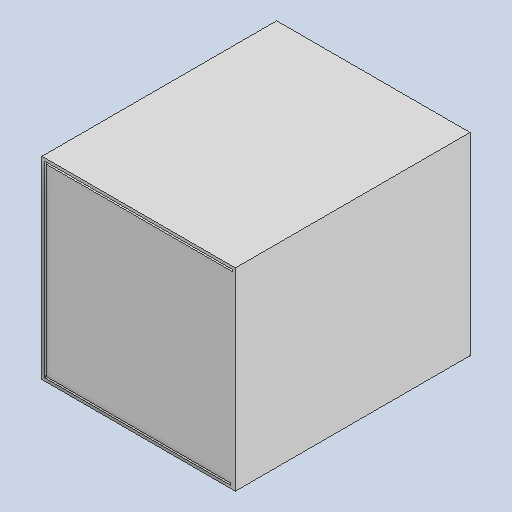
# Autodesk Inventor part: Envolvente
Saved by Autodesk Inventor 2024 (Build 280153000, 153)
## iProperties
Created: 2024-07-16
Part Number: Envolvente
Material: Genérico
Document SubType Name: Modeling
Designer: sergi
Density: 1 g/cm^3
Appearance: Valor por defecto
Author: sergi
Autodesk Inventor part; units mm, degrees
ref_plane "YZ Plane" through (0, 0, 0) normal (1, 0, 0) x (0, 1, 0)
ref_plane "XZ Plane" through (0, 0, 0) normal (0, 1, 0) x (-1, 0, 0)
ref_plane "XY Plane" through (0, 0, 0) normal (0, 0, 1) x (1, 0, 0)
sketch "Boceto1" plane through (0, 0, 0) normal (0, 0, 1) x (1, 0, 0)
  line L0 (-200, -197.9) -> (-200, 0) projected
  line L1 (-198, 0) -> (-198, -197.9) projected
  line L2 (-200, 0) -> (-198, 0) projected
  line L3 (-197.9, 0) -> (0, 0) projected
  line L4 (0, -2) -> (-197.9, -2) projected
  line L5 (0, 0) -> (0, -2) projected
  line L6 (0, -2.1) -> (0, -200) projected
  line L7 (-2, -200) -> (-2, -2.1) projected
  line L8 (0, -200) -> (-2, -200) projected
  line L9 (-2.1, -200) -> (-200, -200) projected
  line L10 (-200, -198) -> (-2.1, -198) projected
  line L11 (-200, -200) -> (-200, -198) projected
  line L12 (-200, -200) -> (0, -200)
  line L13 (0, -200) -> (0, 0)
  line L14 (0, 0) -> (-200, 0)
  line L15 (-200, 0) -> (-200, -200)
  line L16 (0, 0) -> (0, 3)
  line L17 (0, 3) -> (3, 3)
  line L18 (-200, -200) -> (-203, -200)
  line L19 (-203, -200) -> (-203, -203)
  line L20 (-203, -203) -> (3, -203)
  line L21 (3, -203) -> (3, 3)
  line L22 (3, 3) -> (-203, 3)
  line L23 (-203, 3) -> (-203, -203)
  line L24 (-200, -197.9) -> (-198, -197.9) projected
  line L25 (-197.9, 0) -> (-197.9, -2) projected
  line L26 (0, -2.1) -> (-2, -2.1) projected
  line L27 (-2.1, -200) -> (-2.1, -198) projected
  point P0 (-198, -198)
  point P1 (-198, -2)
  point P2 (-2, -2)
  point P3 (-2, -198)
  dimension "espesor" = 3
  dimension "d1" = 3
  dimension "d2" = 3
  dimension "d3" = 3
  constraints: 24 end point, 4 horizontal, 4 parallel, 3 perpendicular, 1 point on line
  measures "espesor" distance of L3.end L16.end
  measures "d1" distance of L16.end L17.end
  measures "d2" distance of L9.end L18.end
  measures "d3" distance of L18.end L19.end
extrude "Extrusión1" add sketch "Boceto1" along normal blind 220 and the other way blind 30 contours L15 L11 L18 L23 L22 L16 L3 L14 L2 L0 | L24 L1 L14 L25 L4 L13 L26 L7 L12 L27 L10 L15 | L9 L12 L8 L6 L13 L5 L16 L17 L21 L20 L19 L18 | L7 L26 L6 L8
equation "\"d1\" = espesor"
equation "\"d2\" = espesor"
equation "\"d3\" = espesor"
